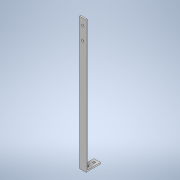
# Autodesk Inventor part: 20220524_知能ロボットカメラ固定部品
Saved by Autodesk Inventor 2020 (Build 240168000, 168)
## iProperties
Created: 2022-05-08
Part Number: 20220524_知能ロボットカメラ固定部品
Material: 一般
Document SubType Name: Modeling
Designer: Naggy
Density: 1 g/cm^3
Appearance: 既定
Author: Naggy
Autodesk Inventor part; units mm, degrees
ref_plane "YZ Plane" through (0, 0, 0) normal (1, 0, 0) x (0, 1, 0)
ref_plane "XZ Plane" through (0, 0, 0) normal (0, 1, 0) x (-1, 0, 0)
ref_plane "XY Plane" through (0, 0, 0) normal (0, 0, 1) x (1, 0, 0)
sketch "スケッチ1" plane through (0, 0, 0) normal (0, 0, 1) x (1, 0, 0)
  line L0 (-5, -100) -> (5, -100)
  line L1 (5, -100) -> (5, 100)
  line L2 (5, 100) -> (-5, 100)
  line L3 (-5, 100) -> (-5, -100)
  line L4 (-5, -100) -> (5, 100) construction
  line L5 (5, -100) -> (-5, 100) construction
  point P0 (0, 0)
  dimension "d0" = 10
  dimension "d1" = 200
  constraints: 12 end point, 2 midpoint, 2 parallel, 1 horizontal, 1 perpendicular
  measures "d0" distance between parallel lines of L1 L3
  measures "d1" distance between parallel lines of L0 L2
extrude "押し出し1" add sketch "スケッチ1" along normal blind 2
sketch "スケッチ2" plane through (0, 0, 2) normal (0, 0, 1) x (1, 0, 0)
  line L0 (5, 100) -> (-5, 100) projected
  point P0 (0, 0)
  point P1 (0, 100)
  point P2 (0, 90)
  point P3 (0, 70)
  dimension "d4" = 10
  dimension "d5" = 20
  constraints: 1 midpoint
  measures "d4" distance from line of point (0, 90) L0
  measures "d5" distance of point (0, 70) point (0, 90)
hole "穴1" at (0, 90, 2) at (0, 70, 2) direction (0, 0, -1) diameter 3.4 end through all clearance for "Flat Head Machine Screw" size "M3" standard "Ansi Metric M Profile"
sketch "スケッチ3" plane through (0, 0, 0) normal (0, 0, -1) x (-1, 0, 0)
  line L0 (5, -100) -> (-5, -100) projected
  line L1 (-5, -100) -> (5, -100)
  line L2 (5, -100) -> (5, -98)
  line L3 (5, -98) -> (-5, -98)
  line L4 (-5, -98) -> (-5, -100)
  point P0 (0, 0)
  dimension "d13" = 2
  constraints: 8 end point, 2 parallel, 1 horizontal, 1 perpendicular
  measures "d13" distance between parallel lines of L3 L0
extrude "押し出し2" add sketch "スケッチ3" along normal blind 20
sketch "スケッチ4" plane through (-5, -98, 0) normal (0, 1, 0) x (1, 0, 0)
  line L0 (0, 20) -> (10, 20) projected
  point P0 (5, 0)
  point P1 (5, 15)
  point P2 (5, 5)
  dimension "d16" = 5
  dimension "d17" = 10
  measures "d16" distance from line of point (5, 15) L0
  measures "d17" distance of point (5, 5) point (5, 15)
hole "穴2" at (0, -98, -15) at (0, -98, -5) direction (0, -1, 0) diameter 3.4 end through all clearance for "Flat Head Machine Screw" size "M3" standard "Ansi Metric M Profile"
